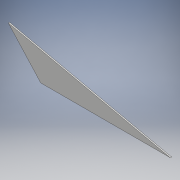
# Autodesk Inventor part: bracket
Saved by Autodesk Inventor 2018.2 (Build 222227000, 227)
## iProperties
Created: 2018-02-26
Part Number: bracket
Material: 一般
Document SubType Name: Modeling
Designer: ku_sk
Density: 1 g/cm^3
Appearance: 既定
Author: ku_sk
Autodesk Inventor part; units mm, degrees
ref_plane "YZ Plane" through (0, 0, 0) normal (1, 0, 0) x (0, 1, 0)
ref_plane "XZ Plane" through (0, 0, 0) normal (0, 1, 0) x (-1, 0, 0)
ref_plane "XY Plane" through (0, 0, 0) normal (0, 0, 1) x (1, 0, 0)
sketch "スケッチ1" plane through (0, 0, 0) normal (0, 1, 0) x (-1, 0, 0)
  line L0 (78, 86) -> (-312, 0)
  line L1 (-312, 0) -> (0, 0)
  line L2 (0, 0) -> (78, 86)
  dimension "d0" = 86
  dimension "d1" = 390
  dimension "d2" = 312
  constraints: 6 end point, 1 coincident, 1 horizontal
  measures "d0" distance from line of L0.start L1
  measures "d1" horizontal distance of L0.end L0.start
  measures "d2" distance of L0.end L1.end
extrude "押し出し1" add sketch "スケッチ1" along normal mid plane 3
